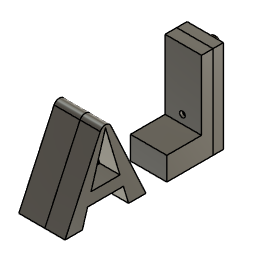
Hardware Exam Practical v8 (Autodesk Fusion 360 design; units mm, degrees)
Autodesk Fusion 360 part; units mm, degrees
sketch "Sketch1" plane through (0, 0, 0) normal (0, 0, 1) x (1, 0, 0)
  line L0 (-25, -50) -> (25, -50)
  line L1 (25, -50) -> (25, 50)
  line L2 (25, 50) -> (-25, 50)
  line L3 (-25, 50) -> (-25, -50)
  line L4 (-25, -50) -> (25, 50) construction
  line L5 (25, -50) -> (-25, 50) construction
  constraint horizontal L0
  constraint perpendicular L0 L1
  constraint parallel L0 L2
  constraint parallel L1 L3
  constraint coincident L4 origin
  constraint coincident L5 origin
sketch "Sketch2" plane through (0, 0, 30) normal (0, 0, 1) x (-1, 0, 0)
  line L0 (25, -50) -> (25, 50)
  line L1 (25, 50) -> (-25, 50)
  line L2 (-25, 50) -> (-25, -50)
  line L3 (-25, -50) -> (25, -50)
  line L4 (25, 15) -> (-25, 15)
  line L5 (-25, 15) -> (-25, 50)
  line L6 (-25, 50) -> (25, 50)
  line L7 (25, 50) -> (25, 15)
  constraint horizontal L4
  constraint vertical L5
  constraint horizontal L6
  constraint vertical L7
  constraint coincident L1.end L2.start
  constraint coincident L0 L4.start
sketch "Sketch3" plane through (0, 0, 0) normal (1, 0, 0) x (0, 1, 0)
  line L0 (100, 0) -> (160, 130)
  line L1 (160, 130) -> (220, 0)
  line L2 (220, 0) -> (190, 0)
  line L3 (190, 0) -> (160, 100)
  line L4 (160, 100) -> (130, 0)
  line L5 (130, 0) -> (100, 0)
  line L6 (139, 30) -> (180, 30)
  line L7 (180, 30) -> (181, 30)
  line L8 (145, 50) -> (175, 50)
  constraint horizontal L2
  constraint parallel L2 L5
  constraint coincident L4 L6.start
  constraint horizontal L6
  constraint coincident L3 L7.end
  constraint parallel L6 L7
  constraint midpoint L4 L8.start
  constraint midpoint L3 L8.end
  constraint parallel L6 L8
extrude "Extrude3" add sketch "Sketch3" along normal blind 60 contours L0 L1 L2 L3 L4 L5 | L3 L4 L6 L7 L8 makes body 1
move_body "Move1" bodies 1 to x (1, 0, 0) y (0, 1, 0) z (0, 0, 1) at (-30, -10, 0)
fillet "Fillet1" radius 10 1 edges at (0, 150, 130) on bodies 1
sketch "Sketch4" plane through (0, 0, 30) normal (0, 0, 1) x (-1, 0, 0)
  line L0 (20, -50) -> (20, 15)
  line L1 (20, 15) -> (-20, 15)
  line L2 (-20, 15) -> (-20, -50)
  line L3 (-20, -50) -> (20, -50)
  circle A0 centre (0, -4) radius 5
move_face "MoveFace1" by (0, -20, 0) 3 faces at (-10, 145, 83.3333) (-10, 126, 20) (-10, 106.9735, 36.7758) on bodies 1
move_face "MoveFace2" by (50, 0, 0) 1 faces at (-30, 105.3068, 60.6647) on bodies 1
copy_body "CopyPasteBodies1" bodies 1 makes body 2
move_body "Move2" bodies 2 to x (1, 0, 0) y (0, 1, 0) z (0, 0, 1) at (-50, 0, 0)
other "Base Mesh Feature1"
other "Modify1"
sketch "Sketch5" plane through (0, 0, 0) normal (0, 0, 1) x (1, 0, 0)
  line L0 (-58, -120) -> (5, -120)
  line L1 (5, -120) -> (5, -40)
  line L2 (5, -40) -> (-58, -40)
  line L3 (-58, -40) -> (-58, -120)
  constraint horizontal L0
  constraint vertical L1
  constraint horizontal L2
  constraint vertical L3
extrude "Extrude5" add sketch "Sketch5" along normal blind 5 separate body makes body 3
sketch "Sketch6" plane through (0, 0, 5) normal (0, 0, 1) x (-1, 0, 0)
  line L0 (58, 40) -> (58, 120)
  line L1 (58, 120) -> (-5, 120)
  line L2 (-5, 120) -> (-5, 40)
  line L3 (-5, 40) -> (58, 40)
  line L4 (58, 40) -> (-5, 40)
  line L5 (-5, 40) -> (-5, 120)
  line L6 (-5, 120) -> (58, 120)
  line L7 (58, 120) -> (58, 40)
  line L8 (55, 43) -> (-3, 43)
  line L9 (-3, 43) -> (-3, 119)
  line L10 (-3, 119) -> (55, 119)
  line L11 (55, 119) -> (55, 43)
  constraint horizontal L4
  constraint vertical L5
  constraint horizontal L6
  constraint vertical L7
  constraint coincident L1.end L2.start
  constraint coincident L0.start L3.end
  constraint horizontal L8
  constraint vertical L9
  constraint horizontal L10
  constraint vertical L11
extrude "Extrude6" add sketch "Sketch6" along normal blind 15 bodies 3
sketch "Sketch7" plane through (0, 0, 20) normal (0, 0, 1) x (-1, 0, 0)
  line L0 (-3, 119) -> (55, 119)
  line L1 (55, 119) -> (55, 43)
  line L2 (55, 43) -> (-3, 43)
  line L3 (-3, 43) -> (-3, 119)
  line L4 (58, 120) -> (-5, 120)
  line L5 (-5, 120) -> (-5, 40)
  line L6 (-5, 40) -> (58, 40)
  line L7 (58, 40) -> (58, 120)
  line L8 (44.5, 119) -> (31.5, 119)
  line L9 (31.5, 119) -> (31.5, 120)
  line L10 (31.5, 120) -> (44.5, 120)
  line L11 (44.5, 120) -> (44.5, 119)
  constraint horizontal L8
  constraint vertical L9
  constraint horizontal L10
  constraint vertical L11
  constraint coincident L4 L9.end
  constraint coincident L0 L8.start
extrude "Extrude7" cut sketch "Sketch7" against normal blind 15 contours L0 L4 L8 L9 L10 L11 bodies 3
other "Modify2"
sketch "Sketch8" plane through (0, 0, 20) normal (0, 0, 1) x (-1, 0, 0)
  line L0 (44.5, 120) -> (44.5, 119)
  line L1 (44.5, 119) -> (55, 119)
  line L2 (55, 119) -> (55, 43)
  line L3 (55, 43) -> (-3, 43)
  line L4 (-3, 43) -> (-3, 119)
  line L5 (-3, 119) -> (31.5, 119)
  line L6 (31.5, 119) -> (31.5, 120)
  line L7 (31.5, 120) -> (-5, 120)
  line L8 (-5, 120) -> (-5, 40)
  line L9 (-5, 40) -> (58, 40)
  line L10 (58, 40) -> (58, 120)
  line L11 (58, 120) -> (44.5, 120)
  line L12 (35, 40) -> (35, 43)
  line L13 (35, 43) -> (55, 43)
  line L14 (55, 43) -> (55, 120)
  line L15 (-5, 120) -> (-5, 43)
  line L16 (20, 43) -> (20, 40)
  line L17 (20, 40) -> (-5, 40)
  line L18 (-5, 43) -> (-5, 40)
  line L19 (35, 40) -> (58, 40)
  line L20 (58, 40) -> (58, 120)
  line L21 (55, 120) -> (58, 120)
  line L22 (55, 120) -> (-5, 120)
  constraint coincident L9 L12.start
  constraint coincident L3 L12.end
  constraint perpendicular L3 L12
  constraint coincident L2.end L3.start
  constraint perpendicular L2 L13
  constraint coincident L11 L14.end
  constraint perpendicular L11 L14
  constraint coincident L7.end L8.start
  constraint coincident L8 L15.end
  constraint coincident L3 L16.start
  constraint coincident L9 L16.end
  constraint perpendicular L9 L16
  constraint coincident L8.end L9.start
  constraint perpendicular L8 L17
  constraint perpendicular L9 L18
  constraint coincident L9.end L10.start
  constraint coincident L10.end L11.start
extrude "Extrude8" add sketch "Sketch8" along normal blind 10 separate body contours L0 L1 L11 L14 L22 | L2 L3 L9 L10 L11 L12 L13 L14 L19 L20 L21 | L3 L4 L5 L6 L7 L8 L9 L15 L16 L17 L18 L22 makes body 4 at (-58, -66.6667, 23.3333) makes body 5 at (5, -93.3333, 23.3333)
sketch "Sketch9" plane through (0, 0, 30) normal (0, 0, 1) x (-1, 0, 0)
  line L0 (35, 40) -> (58, 40)
  line L1 (58, 40) -> (58, 120)
  line L2 (58, 120) -> (55, 120)
  line L3 (55, 120) -> (44.5, 120)
  line L4 (44.5, 120) -> (44.5, 119)
  line L5 (44.5, 119) -> (55, 119)
  line L6 (55, 119) -> (55, 43)
  line L7 (55, 43) -> (35, 43)
  line L8 (35, 43) -> (35, 40)
  line L9 (58, 40) -> (-5, 40)
  line L10 (-5, 40) -> (-5, 120)
  line L11 (-5, 120) -> (58, 120)
  line L12 (58, 120) -> (58, 40)
  constraint horizontal L9
  constraint vertical L10
  constraint horizontal L11
  constraint vertical L12
  constraint coincident L0.end L1.start
extrude "Extrude9" add sketch "Sketch9" along normal blind 5 bodies 4 5
sketch "Sketch10" plane through (0, 0, 0) normal (0, 0, 1) x (1, 0, 0)
  line L0 (5, -40) -> (-58, -40)
  line L1 (-58, -40) -> (-58, 20)
  line L2 (-58, 20) -> (5, 20)
  line L3 (5, 20) -> (5, -40)
  constraint horizontal L0
  constraint vertical L1
  constraint horizontal L2
  constraint vertical L3
extrude "Extrude10" add sketch "Sketch10" along normal blind 20 bodies 3
sketch "Sketch11" plane through (0, 0, 0) normal (0, 0, 1) x (1, 0, 0)
sketch "Sketch12" plane through (0, 0, 20) normal (0, 0, 1) x (-1, 0, 0)
  line L0 (44.5, 120) -> (44.5, 119)
  line L1 (44.5, 119) -> (55, 119)
  line L2 (55, 119) -> (55, 43)
  line L3 (55, 43) -> (-3, 43)
  line L4 (-3, 43) -> (-3, 119)
  line L5 (-3, 119) -> (31.5, 119)
  line L6 (31.5, 119) -> (31.5, 120)
  line L7 (31.5, 120) -> (-5, 120)
  line L8 (-5, 120) -> (-5, -20)
  line L9 (-5, -20) -> (58, -20)
  line L10 (58, -20) -> (58, 120)
  line L11 (58, 120) -> (44.5, 120)
  line L12 (-5, 40.6019) -> (58, 40.6019)
  line L13 (58, 40.6019) -> (58, -20)
  line L14 (58, -20) -> (-5, -20)
  line L15 (-5, -20) -> (-5, 40.6019)
  line L16 (0, 35) -> (55.5, 35)
  line L17 (55.5, 35) -> (55.5, -17.5)
  line L18 (55.5, -17.5) -> (0, -17.5)
  line L19 (0, -17.5) -> (0, 35)
  line L20 (20, 43) -> (35, 43)
  line L21 (35, 43) -> (35, 35)
  line L22 (35, 35) -> (20, 35)
  line L23 (20, 35) -> (20, 43)
  constraint horizontal L12
  constraint vertical L13
  constraint horizontal L14
  constraint vertical L15
  constraint coincident L9.end L10.start
  constraint coincident L8 L12.start
  constraint horizontal L16
  constraint vertical L17
  constraint horizontal L18
  constraint vertical L19
  constraint horizontal L20
  constraint vertical L21
  constraint horizontal L22
  constraint vertical L23
  constraint coincident L16 L21.end
  constraint coincident L3 L20.start
extrude "Extrude11" add sketch "Sketch12" along normal blind 15 contours L8 L9 L10 L12 L13 L14 L15 L16 L17 L18 L19 L21 L23 bodies 4
sketch "Sketch13" plane through (0, 0, 0) normal (0, 0, 1) x (1, 0, 0)
  line L0 (-58, -120) -> (5, -120)
  line L1 (5, -120) -> (5, -80)
  line L2 (5, -80) -> (-58, -80)
  line L3 (-58, -80) -> (-58, -120)
  constraint horizontal L0
  constraint vertical L1
  constraint horizontal L2
  constraint vertical L3
extrude "Extrude12" add sketch "Sketch13" against normal blind 100 bodies 3
other "Base Mesh Feature2"
other "Base Mesh Feature3"
other "CopyPasteMeshes1"
other "Modify3"
other "CopyPasteMeshes2"
other "Modify4"
other "Modify5"
move_face "MoveFace3" by (0, 20, 0) 3 faces at (-37, 17.5, 30) (-37, 20, 13.3333) (-16, 20, 25) on bodies 3 4
other "Modify6"
sketch "Sketch14" plane through (0, 0, 35) normal (0, 0, 1) x (-1, 0, 0)
  line L0 (58, -40) -> (58, 120)
  line L1 (58, 120) -> (-5, 120)
  line L2 (-5, 120) -> (-5, -40)
  line L3 (-5, -40) -> (58, -40)
  line L4 (35, 40) -> (35, 35)
  line L5 (35, 35) -> (55.5, 35)
  line L6 (55.5, 35) -> (55.5, -37.5)
  line L7 (55.5, -37.5) -> (0, -37.5)
  line L8 (0, -37.5) -> (0, 35)
  line L9 (0, 35) -> (20, 35)
  line L10 (20, 35) -> (20, 40)
  line L11 (20, 40) -> (35, 40)
  line L12 (0, 35) -> (55.5, 35)
  line L13 (55.5, 35) -> (55.5, -37.5)
  line L14 (55.5, -37.5) -> (0, -37.5)
  line L15 (0, -37.5) -> (0, 35)
  circle A0 centre (17, 28) radius 2.2361
  circle A1 centre (26.8, 28) radius 2.1108
  circle A2 centre (36.84, 28) radius 2.0834
  circle A3 centre (27.6243, -18.4965) radius 13.6333
  constraint horizontal L12
  constraint vertical L13
  constraint horizontal L14
  constraint vertical L15
  constraint coincident L6.end L7.start
  constraint coincident L8.end L9.start
extrude "Extrude13" add sketch "Sketch14" along normal blind 3 contours L0 L1 L2 L3 | L5 L6 L7 L8 L9 L12 L13 L14 L15 bodies 4
other "Modify7"
move_face "MoveFace4" by (0, -5, 0) 1 faces at (-25, -35, 36) on bodies 4
sketch "Sketch15" plane through (0, 0, 0) normal (0, 0, -1) x (1, 0, 0)
  line L0 (5, 80) -> (-58, 80)
  line L1 (-58, 80) -> (-58, -40)
  line L2 (-58, -40) -> (5, -40)
  line L3 (5, -40) -> (5, 80)
  circle A0 centre (-25, 65) radius 5
extrude "Extrude14" cut sketch "Sketch15" against normal blind 10 contours A0 bodies 3
move_face "MoveFace5" by (0, 0, 40) 1 faces at (-37, -93.3333, -100) on bodies 3
other "Base Mesh Feature4"
other "Modify8"
other "Modify9"
move_body "Move3" bodies 1 2 to x (1, 0, 0) y (0, 1, 0) z (0, 0, 1) at (0, 5, 0)
move_body "Move4" bodies 1 to x (1, 0, 0) y (0, 1, 0) z (0, 0, 1) at (10, 0, 0)
move_body "Move5" bodies 2 to x (1, 0, 0) y (0, 1, 0) z (0, 0, 1) at (-5, 0, 0)
move_body "Move6" bodies 1 to x (1, 0, 0) y (0, 1, 0) z (0, 0, 1) at (-5, 0, 0)
sketch "Sketch16" plane through (-25, 0, 0) normal (1, 0, 0) x (0, 1, 0)
  arc A0 (154.0796, 131.9942) -> (135.9204, 131.9942) centre (145, 127.8036) ccw
  line L0 (135.9204, 131.9942) -> (75, 0)
  line L1 (75, 0) -> (105, 0)
  line L2 (105, 0) -> (114, 30)
  line L3 (114, 30) -> (176, 30)
  line L4 (176, 30) -> (185, 0)
  line L5 (185, 0) -> (215, 0)
  line L6 (215, 0) -> (154.0796, 131.9942)
  line L7 (170, 50) -> (120, 50)
  line L8 (120, 50) -> (145, 133.3333)
  line L9 (145, 133.3333) -> (170, 50)
  line L10 (170, 48) -> (118, 48)
  line L11 (118, 48) -> (118, 33)
  line L12 (118, 33) -> (171, 33)
  line L13 (171, 33) -> (171, 48)
  line L14 (171, 48) -> (170, 48)
  constraint horizontal L10
  constraint perpendicular L10 L11
  constraint perpendicular L11 L12
  constraint perpendicular L12 L13
  constraint perpendicular L13 L14
extrude "Extrude15" cut sketch "Sketch16" against normal blind 10 contours L10 L11 L12 L13 L14 bodies 2
extrude "Extrude16" add 1 faces at (-25, 179.6932, 60.6647) along direction (1, 0, 0) blind 30 on bodies 2 bodies 2
other "Modify10"
sketch "Sketch17" plane through (0, 171, 0) normal (0, -1, 0) x (1, 0, 0)
  line L0 (5, 48) -> (-35, 48)
  line L1 (-35, 48) -> (-35, 33)
  line L2 (-35, 33) -> (5, 33)
  line L3 (5, 33) -> (5, 48)
  circle A0 centre (-25, 40) radius 5
extrude "Extrude17" add sketch "Sketch17" along normal blind 30 contours A0 bodies 2
sketch "Sketch18" plane through (-35, 0, 0) normal (-1, 0, 0) x (0, -1, 0)
  line L0 (-118, 48) -> (-118, 33)
  line L1 (-118, 33) -> (-171, 33)
  line L2 (-171, 33) -> (-171, 48)
  line L3 (-171, 48) -> (-118, 48)
  line L4 (-120, 50) -> (-170, 50)
  line L5 (-170, 50) -> (-145, 133.3333)
  line L6 (-145, 133.3333) -> (-120, 50)
  arc A0 (-135.9204, 131.9942) -> (-154.0796, 131.9942) centre (-145, 127.8036) ccw
  line L7 (-154.0796, 131.9942) -> (-215, 0)
  line L8 (-215, 0) -> (-185, 0)
  line L9 (-185, 0) -> (-176, 30)
  line L10 (-176, 30) -> (-114, 30)
  line L11 (-114, 30) -> (-105, 0)
  line L12 (-105, 0) -> (-75, 0)
  line L13 (-75, 0) -> (-135.9204, 131.9942)
  line L14 (-118, 48) -> (-171, 48)
  line L15 (-171, 48) -> (-171, 33)
  line L16 (-171, 33) -> (-118, 33)
  line L17 (-118, 33) -> (-118, 48)
  constraint horizontal L14
  constraint vertical L15
  constraint horizontal L16
  constraint vertical L17
  constraint coincident L1.end L2.start
  constraint coincident L0.start L3.end
extrude "Extrude18" add sketch "Sketch18" along normal blind 5 separate body contours L0 L1 L2 L3 L14 L15 L16 L17 makes body 6
sketch "Sketch19" plane through (-35, 0, 0) normal (-1, 0, 0) x (0, -1, 0)
  line L0 (-118, 48) -> (-118, 33)
  line L1 (-118, 33) -> (-171, 33)
  line L2 (-171, 33) -> (-171, 48)
  line L3 (-171, 48) -> (-118, 48)
  line L4 (-120, 50) -> (-170, 50)
  line L5 (-170, 50) -> (-145, 133.3333)
  line L6 (-145, 133.3333) -> (-120, 50)
  arc A0 (-135.9204, 131.9942) -> (-154.0796, 131.9942) centre (-145, 127.8036) ccw
  line L7 (-154.0796, 131.9942) -> (-215, 0)
  line L8 (-215, 0) -> (-185, 0)
  line L9 (-185, 0) -> (-176, 30)
  line L10 (-176, 30) -> (-114, 30)
  line L11 (-114, 30) -> (-105, 0)
  line L12 (-105, 0) -> (-75, 0)
  line L13 (-75, 0) -> (-135.9204, 131.9942)
extrude "Extrude19" add sketch "Sketch19" along normal blind 5 bodies 2 6
sketch "Sketch20" plane through (0, 0, 50) normal (0, 0, 1) x (-1, 0, 0)
  line L0 (40, -120) -> (-5, -120)
  line L1 (-5, -120) -> (-5, -170)
  line L2 (-5, -170) -> (40, -170)
  line L3 (40, -170) -> (40, -120)
  circle A0 centre (3, -143) radius 7
extrude "Extrude20" cut sketch "Sketch20" against normal blind 5 contours A0 bodies 2
sketch "Sketch21" plane through (25, 0, 0) normal (-1, 0, 0) x (0, -1, 0)
  line L0 (-120, 50) -> (-170, 50)
  line L1 (-170, 50) -> (-145, 133.3333)
  line L2 (-145, 133.3333) -> (-120, 50)
  arc A0 (-135.9204, 131.9942) -> (-154.0796, 131.9942) centre (-145, 127.8036) ccw
  line L3 (-154.0796, 131.9942) -> (-215, 0)
  line L4 (-215, 0) -> (-185, 0)
  line L5 (-185, 0) -> (-176, 30)
  line L6 (-176, 30) -> (-114, 30)
  line L7 (-114, 30) -> (-105, 0)
  line L8 (-105, 0) -> (-75, 0)
  line L9 (-75, 0) -> (-135.9204, 131.9942)
  line L10 (-171, 48) -> (-120, 48)
  line L11 (-120, 48) -> (-120, 33)
  line L12 (-120, 33) -> (-171, 33)
  line L13 (-171, 33) -> (-171, 48)
  constraint horizontal L10
  constraint vertical L11
  constraint horizontal L12
  constraint vertical L13
extrude "Extrude21" cut sketch "Sketch21" against normal blind 8 contours L10 L11 L12 L13 bodies 1
extrude "Extrude22" add 1 faces at (35, 110.3068, 60.6647) along direction (1, 0, 0) blind 5 on bodies 1 bodies 1
extrude "Extrude23" cut 1 faces at (33, 154, 43) along direction (1, 0, 0) blind 3 on bodies 1 bodies 1
extrude "Extrude24" add 1 faces at (25, 110.3068, 60.6647) along direction (-1, 0, 0) blind 20 on bodies 1 bodies 1
move_body "Move7" bodies 3 4 to x (-1, 0, 0) y (0, 0, 1) z (0, 1, 0) at (-23.34, 316.57, 113.43)
other "Modify11"
copy_body "Body->Comp1" bodies 4 removing the originals makes body 7 in component "LGun Top"
copy_body "Body->Comp2" bodies 3 removing the originals makes body 8 in component "LGun Bottom"
other "Body->Comp1'"
other "Body->Comp2'"
other "Body->Comp3"
other "Body->Comp4"
other "Body->Comp5"
copy_body "Body->Comp3'" bodies 1 removing the originals makes body 9 in component "ABack"
copy_body "Body->Comp4'" bodies 2 removing the originals makes body 10 in component "AFront"
other "Body->Comp6"
component "LGun Top" placed x (1, 0, 0) y (0, 1, 0) z (0, 0, 1) at (0, 0, 0)
component "LGun Bottom" placed x (1, 0, 0) y (0, 1, 0) z (0, 0, 1) at (0, 0, 0)
component "ARDUINO-UNO_20 v1" placed x (1, 0, 0) y (0, 1, 0) z (0, 0, 1) at (0, 0, 0)
component "Joystick v1" placed x (1, 0, 0) y (0, 1, 0) z (0, 0, 1) at (0, 0, 0)
component "LED1 v1" placed x (1, 0, 0) y (0, 1, 0) z (0, 0, 1) at (0, 0, 0)
component "LED2" placed x (1, 0, 0) y (0, 1, 0) z (0, 0, 1) at (0, 0, 0)
component "LED3" placed x (1, 0, 0) y (0, 1, 0) z (0, 0, 1) at (0, 0, 0)
component "ABack" placed x (1, 0, 0) y (0, 1, 0) z (0, 0, 1) at (0, 0, 0)
component "AFront" placed x (1, 0, 0) y (0, 1, 0) z (0, 0, 1) at (0, 0, 0)
component "Micro:Bit" placed x (1, 0, 0) y (0, 1, 0) z (0, 0, 1) at (0, 0, 0)
